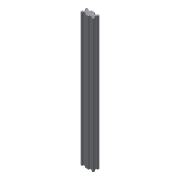
# Autodesk Inventor part: 20X40long
Saved by Autodesk Inventor 2015 SP1 (Build 190203100, 203)
## iProperties
Created: 2015-01-22
Part Number: 20X40long
Material: Aluminum 6061
Document SubType Name: Modeling
Designer: rihoobler
Density: 2.7 g/cm^3
Appearance: Aluminum - Flat
Author: rihoobler
Autodesk Inventor part; units mm, degrees
ref_plane "YZ Plane" through (0, 0, 0) normal (1, 0, 0) x (0, 1, 0)
ref_plane "XZ Plane" through (0, 0, 0) normal (0, 1, 0) x (-1, 0, 0)
sketch "Sketch1" plane through (0, 0, 0) normal (0, 1, 0) x (-1, 0, 0)
  line L0 (0, 0) -> (40, 0)
  line L1 (40, 0) -> (40, 20)
  line L2 (40, 20) -> (0, 20)
  line L3 (0, 20) -> (0, 0)
  line L4 (0, 14) -> (4, 14)
  line L5 (4, 14) -> (4, 6)
  line L6 (4, 6) -> (0, 6)
  line L7 (0, 6) -> (0, 14)
  line L8 (40, 14) -> (36, 14)
  line L9 (36, 14) -> (36, 6)
  line L10 (36, 6) -> (40, 6)
  line L11 (40, 6) -> (40, 14)
  line L12 (6, 0) -> (14, 0)
  line L13 (14, 0) -> (14, 4)
  line L14 (14, 4) -> (6, 4)
  line L15 (6, 4) -> (6, 0)
  line L16 (26, 0) -> (34, 0)
  line L17 (34, 0) -> (34, 4)
  line L18 (34, 4) -> (26, 4)
  line L19 (26, 4) -> (26, 0)
  line L20 (6, 20) -> (14, 20)
  line L21 (14, 20) -> (14, 16)
  line L22 (14, 16) -> (6, 16)
  line L23 (6, 16) -> (6, 20)
  line L24 (26, 20) -> (34, 20)
  line L25 (34, 20) -> (34, 16)
  line L26 (34, 16) -> (26, 16)
  line L27 (26, 16) -> (26, 20)
  dimension "d0" = 40
  dimension "d1" = 20
  dimension "d2" = 6
  dimension "d3" = 8
  dimension "d4" = 4
  dimension "d5" = 8
  dimension "d6" = 6
  dimension "d7" = 4
  dimension "d8" = 4
  dimension "d9" = 8
  dimension "d10" = 6
  dimension "d11" = 4
  constraints: 56 end point, 14 parallel, 14 point on line, 7 horizontal, 7 perpendicular
  measures "d0" distance of L2.end L1.end
  measures "d1" distance of L1.end L0.end
  measures "d2" distance between parallel lines of L2 L4
  measures "d3" distance between parallel lines of L6 L4
  measures "d4" distance of L5.end L6.end
  measures "d5" distance between parallel lines of L13 L15
  measures "d6" distance between parallel lines of L3 L15
  measures "d7" distance between parallel lines of L0 L14
  measures "d8" distance between parallel lines of L2 L22
  measures "d9" distance between parallel lines of L17 L19
  measures "d10" distance between parallel lines of L1 L17
  measures "d11" distance of L9.end L10.end
extrude "Extrusion1" add sketch "Sketch1" along normal blind 413.004 contours L3 L6 L5 L4 L2 L23 L22 L21 L27 L26 L25 L1 L8 L9 L10 L0 L17 L18 L19 L13 L14 L15
fillet "Fillet1" radius 1.27 16 edges at (-40, 206.502, 20) (-40, 206.502, 14) (-40, 206.502, 6) (-40, 206.502, 0) (-34, 206.502, 0) (-34, 206.502, 20) (-26, 206.502, 20) (-14, 206.502, 20) (-6, 206.502, 20) (0, 206.502, 20) (0, 206.502, 14) (0, 206.502, 6) (0, 206.502, 0) (-6, 206.502, 0) (-14, 206.502, 0) (-26, 206.502, 0)
ref_plane "Work Plane1" through (-24.73, 0, 10) normal (0, 0, 1) x (1, 0, 0)
body "Solid1"
